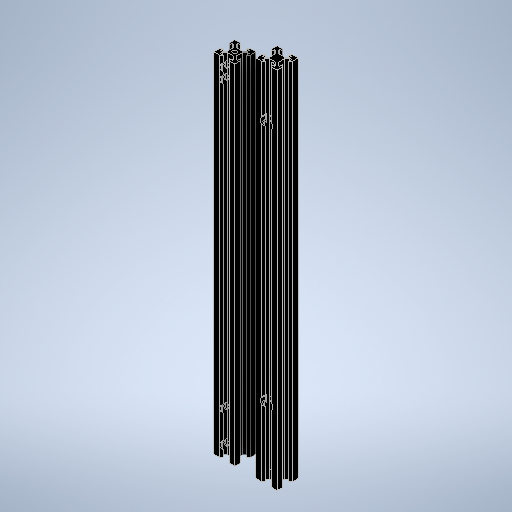
# Autodesk Inventor part: 2020 Extrusions
Saved by Autodesk Inventor 2025 (Build 290162000, 162)
## iProperties
Created: 2025-01-25
Part Number: 2020 Extrusions
Material: Aluminum 6061
Document SubType Name: Modeling
Designer: rdmal
Density: 2.7 g/cm^3
Appearance: Anodized - Black
Mass: 156.508 g
Surface Area: 533.582 cm^2
Volume: 57.966 cm^3
Author: rdmal
Autodesk Inventor part; units mm, degrees
ref_plane "YZ Plane" through (0, 0, 0) normal (1, 0, 0) x (0, 1, 0)
sketch "Sketch1" plane through (0, 0, 0) normal (0, 1, 0) x (-1, 0, 0)
  circle A0 centre (0, 0) radius 2.1
  line L0 (3.1, -4.1607) -> (-3.1, -4.1607)
  line L1 (3.1, 4.1607) -> (-3.1, 4.1607)
  line L2 (4.1607, -3.1) -> (4.1607, 3.1)
  line L3 (-4.1607, -3.1) -> (-4.1607, 3.1)
  line L4 (14, 0) -> (-14, 0) projected
  line L5 (0, -14) -> (0, 14) projected
  line L6 (4.1607, -3.1) -> (6.5607, -5.5)
  line L7 (3.1, -4.1607) -> (5.5, -6.5607)
  line L8 (-3.1, -4.1607) -> (-5.5, -6.5607)
  line L9 (-4.1607, -3.1) -> (-6.5607, -5.5)
  line L10 (4.1607, 3.1) -> (6.5607, 5.5)
  line L11 (3.1, 4.1607) -> (5.5, 6.5607)
  line L12 (-3.1, 4.1607) -> (-5.5, 6.5607)
  line L13 (-4.1607, 3.1) -> (-6.5607, 5.5)
  line L14 (5.5, -6.5607) -> (5.5, -8.2)
  line L15 (-5.5, -6.5607) -> (-5.5, -8.2)
  line L16 (6.5607, -5.5) -> (8.2, -5.5)
  line L17 (6.5607, 5.5) -> (8.2, 5.5)
  line L18 (5.5, 6.5607) -> (5.5, 8.2)
  line L19 (-5.5, 6.5607) -> (-5.5, 8.2)
  line L20 (-6.5607, 5.5) -> (-8.2, 5.5)
  line L21 (-6.5607, -5.5) -> (-8.2, -5.5)
  line L22 (5.5, -8.2) -> (2.975, -8.2)
  line L23 (-5.5, -8.2) -> (-2.975, -8.2)
  line L24 (-8.2, -5.5) -> (-8.2, -2.975)
  line L25 (-8.2, 5.5) -> (-8.2, 2.975)
  line L26 (-5.5, 8.2) -> (-2.975, 8.2)
  line L27 (5.5, 8.2) -> (2.975, 8.2)
  line L28 (8.2, 5.5) -> (8.2, 2.975)
  line L29 (8.2, -5.5) -> (8.2, -2.975)
  line L30 (2.975, -8.2) -> (4.775, -10)
  line L31 (-2.975, -8.2) -> (-4.775, -10)
  line L32 (-8.2, -2.975) -> (-10, -4.775)
  line L33 (-8.2, 2.975) -> (-10, 4.775)
  line L34 (-2.975, 8.2) -> (-4.775, 10)
  line L35 (2.975, 8.2) -> (4.775, 10)
  line L36 (8.2, 2.975) -> (10, 4.775)
  line L37 (8.2, -2.975) -> (10, -4.775)
  line L38 (10, -4.775) -> (10, -10)
  line L39 (10, -10) -> (4.775, -10)
  line L40 (-4.775, -10) -> (-10, -10)
  line L41 (-10, -10) -> (-10, -4.775)
  line L42 (-10, 4.775) -> (-10, 10)
  line L43 (-10, 10) -> (-4.775, 10)
  line L44 (4.775, 10) -> (10, 10)
  line L45 (10, 10) -> (10, 4.775)
  point P0 (4.1607, 0)
  point P1 (0, -4.1607)
  point P2 (-4.1607, 0)
  point P3 (0, 4.1607)
  dimension "d80" = 4.2
  dimension "d83" = 1.5
  dimension "d84" = 90
  dimension "d85" = 1.8
  dimension "d86" = 20
  dimension "d87" = 20
  dimension "d88" = 11
  dimension "d90" = 9.55
  dimension "d91" = 6.2
  constraints: 88 end point, 38 equal length, 12 horizontal, 11 vertical, 7 point on line, 6 midpoint, 4 parallel, 4 perpendicular, 2 collinear, 1 centre point
  measures "d80" diameter of A0
  measures "d83" distance between parallel lines of L9 L8
  measures "d84" angle of L31 L30
  measures "d85" distance between parallel lines of L40 L23
  measures "d86" distance between parallel lines of L44 L39
  measures "d87" distance between parallel lines of L42 L45
  measures "d88" distance between parallel lines of L19 L18
  measures "d90" distance of L31.end L30.end
  measures "d91" distance of L0.start L0.end
extrude "Extrusion2" add sketch "Sketch1" along normal blind 330 contours L4 L2 L6 L16 L29 L37 L38 L39 L30 L22 L14 L7 L0 L5 A0 | A0 L5 L1 L11 L18 L27 L35 L44 L45 L36 L28 L17 L10 L2 L4 | A0 L4 L3 L13 L20 L25 L33 L42 L43 L34 L26 L19 L12 L1 L5 | L5 L0 L8 L15 L23 L31 L40 L41 L32 L24 L21 L9 L3 L4 A0
extrude "Extrusion3" add sketch "Sketch1" along normal blind 345 separate body
move or copy body "Move Body2" bodies to move or copy 2 copy no translate (40, 0, 0)
ref_plane "Work Plane1" through (47.3875, 345, 10) normal (0, 0, 1) x (1, 0, 0)
sketch "Sketch4" plane through (47.3875, 345, 10) normal (0, 0, 1) x (1, 0, 0)
  line L0 (-10.4875, 0) -> (-4.2875, 0) projected
  line L1 (-7.3875, 0) -> (-7.3875, -345) construction
  line L2 (-10.4875, -345) -> (-4.2875, -345) projected
  point P0 (-47.3875, -345)
  point P1 (-7.3875, -3)
  point P2 (-7.3875, -29)
  point P3 (-7.3875, -256.7)
  point P4 (-7.3875, -336.4)
  point P5 (-7.3875, -48.6)
  point P6 (-7.3875, -278.8)
  dimension "d116" = 3
  dimension "d117" = 29
  dimension "d118" = 256.7
  dimension "d119" = 336.4
  dimension "d120" = 48.6
  dimension "d121" = 278.8
  constraints: 6 point on line, 2 end point, 2 midpoint
  measures "d116" distance from line of L0 point (-7.387, -3)
  measures "d117" distance from line of L0 point (-7.387, -29)
  measures "d118" distance from line of L0 point (-7.387, -256.7)
  measures "d119" distance from line of L0 point (-7.387, -336.4)
  measures "d120" distance from line of L0 point (-7.387, -48.6)
  measures "d121" distance from line of L0 point (-7.387, -278.8)
hole "Hole2" at (40, 342, 10) at (40, 316, 10) at (40, 8.6, 10) at (40, 88.3, 10) direction (0, 0, -1) diameter 3.3 end through all bodies 2
hole "Hole3" at (40, 296.4, 10) at (40, 66.2, 10) direction (0, 0, -1) diameter 6 end through all counterbore diameter 11.5 counterbore depth 4.5 bodies 2
ref_plane "Work Plane2" through (7.3875, 330, 10) normal (0, 0, 1) x (1, 0, 0)
sketch "Sketch5" plane through (7.3875, 330, 10) normal (0, 0, 1) x (1, 0, 0)
  line L0 (-10.4875, 0) -> (-4.2875, 0) construction
  line L1 (-7.3875, 0) -> (-7.3875, -330) construction
  point P0 (-7.3875, -10)
  point P1 (-7.3875, -20)
  point P2 (-7.3875, -290)
  point P3 (-7.3875, -320)
  dimension "d136" = 310
  dimension "d137" = 10
  dimension "d138" = 20
  dimension "d139" = 270
  constraints: 4 point on line, 2 end point, 1 midpoint, 1 vertical
  measures "d136" distance of point (-7.388, -320) point (-7.388, -10)
  measures "d137" distance from line of L0 point (-7.388, -10)
  measures "d138" distance from line of L0 point (-7.388, -20)
  measures "d139" distance of point (-7.388, -20) point (-7.388, -290)
hole "Hole4" at (0, 320, 10) at (0, 310, 10) at (0, 40, 10) at (0, 10, 10) direction (0, 0, -1) diameter 5.2 end through all counterbore diameter 9.5 counterbore depth 5.8 bodies 1
